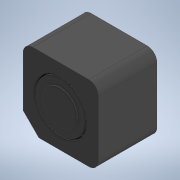
# Autodesk Inventor part: Деталь1
Saved by Autodesk Inventor 2020 (Build 240168000, 168)
## iProperties
Created: 2020-02-28
Part Number: Деталь1
Material: Типовые
Document SubType Name: Modeling
Designer: Andre
Density: 1 g/cm^3
Appearance: По умолчанию
Author: Andre
Autodesk Inventor part; units mm, degrees
ref_plane "YZ Plane" through (0, 0, 0) normal (1, 0, 0) x (0, 1, 0)
ref_plane "XZ Plane" through (0, 0, 0) normal (0, 1, 0) x (-1, 0, 0)
ref_plane "XY Plane" through (0, 0, 0) normal (0, 0, 1) x (1, 0, 0)
sketch "Эскиз1" plane through (0, 0, 0) normal (0, 0, 1) x (1, 0, 0)
  line L0 (-3.1, 3.1) -> (3.1, 3.1)
  line L1 (3.1, 3.1) -> (3.1, -3.1)
  line L2 (3.1, -3.1) -> (-3.1, -3.1)
  line L3 (-3.1, -3.1) -> (-3.1, 3.1)
  line L4 (-3.1, 3.1) -> (3.1, -3.1) construction
  line L5 (3.1, 3.1) -> (-3.1, -3.1) construction
  point P0 (0, 0)
  dimension "d0" = 6.2
  dimension "d1" = 6.2
  constraints: 12 end point, 2 midpoint, 2 parallel, 1 horizontal, 1 perpendicular
  measures "d0" distance of L1.end L2.end
  measures "d1" distance of L0.end L1.end
extrude "Выдавливание1" add sketch "Эскиз1" along normal blind 4.8
fillet "Сопряжение1" radius 0.8 3 edges at (3.1, 3.1, 2.4) (3.1, -3.1, 2.4) (-3.1, 3.1, 2.4)
chamfer "Фаска1" distance 1.3 angle 45 1 edges at (-3.1, -3.1, 2.4)
sketch "Эскиз2" plane through (0, 0, 4.8) normal (0, 0, 1) x (1, 0, 0)
  circle A0 centre (0, 0) radius 2.05
  circle A1 centre (0, 0) radius 2.15
  dimension "d9" = 4.3
  constraints: 2 centre point, 2 coincident
  measures "d9" diameter of A1
extrude "Выдавливание2" cut sketch "Эскиз2" against normal blind 4 contours A0 | A1
sketch "Эскиз3" plane through (0, 0, 0.8) normal (0, 0, 1) x (1, 0, 0)
  circle A0 centre (0, 0) radius 2.05
  dimension "d12" = 4.1
  constraints: 1 centre point, 1 coincident
  measures "d12" diameter of A0
extrude "Выдавливание3" add sketch "Эскиз3" along normal blind 4
sketch "Эскиз4" plane through (0, 0, 4.8) normal (0, 0, 1) x (1, 0, 0)
  circle A0 centre (0, 0) radius 1.4
  dimension "d15" = 2.8
  constraints: 1 centre point, 1 coincident
  measures "d15" diameter of A0
extrude "Выдавливание4" add sketch "Эскиз4" along normal blind 0.1
sketch "Эскиз5" plane through (0, 0, 0) normal (0, 0, -1) x (-1, 0, 0)
  line L0 (-1.6, -1) -> (-2.6, -1)
  line L1 (-2.6, -1) -> (-2.6, 1)
  line L2 (-2.6, 1) -> (-1.6, 1)
  line L3 (-1.6, 1) -> (-1.6, -1)
  line L4 (-1.6, -1) -> (-2.6, 1) construction
  line L5 (-2.6, -1) -> (-1.6, 1) construction
  line L6 (1.6, -1) -> (2.6, -1)
  line L7 (2.6, -1) -> (2.6, 1)
  line L8 (2.6, 1) -> (1.6, 1)
  line L9 (1.6, 1) -> (1.6, -1)
  line L10 (1.6, -1) -> (2.6, 1) construction
  line L11 (2.6, -1) -> (1.6, 1) construction
  point P0 (0, 0)
  dimension "d28" = 1
  dimension "d29" = 2
  dimension "d31" = 1
  dimension "d32" = 2
  constraints: 24 end point, 4 parallel, 2 horizontal, 2 perpendicular
  measures "d28" distance of L1.end L2.end
  measures "d29" distance of L1.end L0.end
  measures "d31" distance of L8.end L7.end
  measures "d32" distance of L7.end L6.end
extrude "Выдавливание5" add sketch "Эскиз5" along normal blind 0.1
